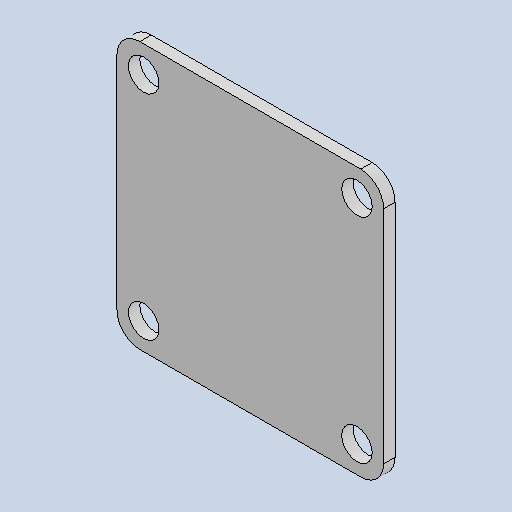
# Autodesk Inventor part: GNH 018  Plate pulse pillar
Saved by Autodesk Inventor 2025.1 (Build 291241020, 241B)
## iProperties
Created: 2023-03-28
Part Number: GNH 018  Plate pulse pillar
Material: Stainless Steel
Description: bend
Document SubType Name: Sheet Metal
Designer: user
Stock Number: bend
Mass: 112.033 g
Surface Area: 104.468 cm^2
Volume: 14.0041 cm^3
Density: 8 g/cm^3
Flat Pattern Width: 7 cm
Flat Pattern Length: 7 cm
Flat Pattern Area: 49 cm^2
Sheet Metal Rule: Default_mm
Sheet Metal Width: 70.000 mm
Sheet Metal Length: 70.000 mm
Sheet Metal Area: 4900.000 mm^2
Appearance: Default
Author: user
Autodesk Inventor part; units mm, degrees
ref_plane "YZ Plane" through (0, 0, 0) normal (1, 0, 0) x (0, 1, 0)
ref_plane "XZ Plane" through (0, 0, 0) normal (0, 1, 0) x (-1, 0, 0)
ref_plane "XY Plane" through (0, 0, 0) normal (0, 0, 1) x (1, 0, 0)
sketch "Sketch1" plane through (0, 0, 0) normal (0, 0, 1) x (1, 0, 0)
  line L0 (35, -35) -> (-35, -35)
  line L1 (-35, -35) -> (-35, 35)
  line L2 (-35, 35) -> (35, 35)
  line L3 (35, 35) -> (35, -35)
  line L4 (35, 35) -> (-35, -35) construction
  point P0 (0, 0)
  point P1 (0, 0)
  dimension "d1" = 70
  dimension "d2" = 70
  constraints: 10 end point, 2 parallel, 1 coincident, 1 horizontal, 1 midpoint, 1 perpendicular
  measures "d1" distance of L2.end L0.start
  measures "d2" distance of L1.end L2.end
extrude "Plate1" add sketch "Sketch1" along normal blind 3
sketch "Sketch2" plane through (0, 0, 0) normal (0, 0, 1) x (1, 0, 0)
  line L0 (28, -28) -> (-28, -28) construction
  line L1 (-28, -28) -> (-28, 28) construction
  line L2 (-28, 28) -> (28, 28) construction
  line L3 (28, 28) -> (28, -28) construction
  line L4 (28, -28) -> (-28, 28) construction
  line L5 (-28, -28) -> (28, 28) construction
  circle A0 centre (-28, -28) radius 4
  circle A1 centre (28, -28) radius 4
  circle A2 centre (28, 28) radius 4
  circle A3 centre (-28, 28) radius 4
  line L6 (28, 0) -> (-28, 0) construction
  line L7 (-20, 20) -> (20, 20) construction
  line L8 (20, 20) -> (20, -20) construction
  line L9 (20, -20) -> (-20, -20) construction
  line L10 (-20, -20) -> (-20, 20) construction
  line L11 (-20, 20) -> (20, -20) construction
  line L12 (20, 20) -> (-20, -20) construction
  line L13 (-35, -35) -> (-35, 35) projected
  line L14 (35, -35) -> (-35, -35) projected
  line L15 (35, 35) -> (35, -35) projected
  line L16 (-35, 35) -> (35, 35) projected
  point P0 (0, 0)
  point P1 (75, 0)
  point P2 (0, 0)
  dimension "d7" = 8
  dimension "d33" = 40
  dimension "d35" = 7
  constraints: 26 end point, 5 coincident, 5 midpoint, 4 centre point, 4 parallel, 3 equal radius, 2 horizontal, 2 perpendicular, 1 point on line
  measures "d7" diameter of A0
  measures "d33" distance of L7.start L7.end
  measures "d35" distance from line of L13 L1.end
extrude "Extrusion1" cut sketch "Sketch2" along normal through all contours A0 | A1 | A2 | A3
fillet "Corner Round1" radius 6 4 edges at (-35, 35, 1.5) (35, 35, 1.5) (35, -35, 1.5) (-35, -35, 1.5)
equation "\"d1\" = d2"
equation "\"d0\" = Thickness"
equation "\"BendRadius\" = Thickness"
equation "\"BendReliefWidth\" = Thickness"
equation "\"BendReliefDepth\" = 0.5 * Thickness"
equation "\"CornerReliefSize\" = 4 * Thickness"
equation "\"MinimumRemnant\" = 2 * Thickness"
equation "\"TransitionRadius\" = BendRadius"
equation "\"JacobiRadiusSize\" = BendRadius"
equation "\"GapSize\" = Thickness"
equation "\"Thickness\" = 3"
body "Solid1"
